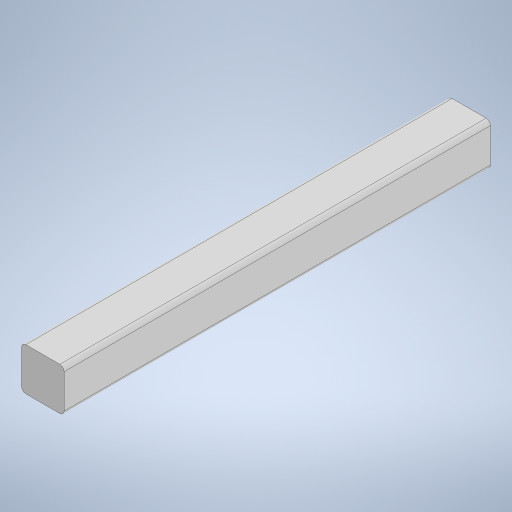
# Autodesk Inventor part: MagnetShaft
Saved by Autodesk Inventor 2024.4 (Build 284460000, 460)
## iProperties
Created: 2025-12-17
Part Number: MagnetShaft
Material: Generic
Document SubType Name: Modeling
Designer: jonas
Density: 1 g/cm^3
Appearance: Default
Author: jonas
Autodesk Inventor part; units mm, degrees
ref_plane "YZ Plane" through (0, 0, 0) normal (1, 0, 0) x (0, 1, 0)
ref_plane "XZ Plane" through (0, 0, 0) normal (0, 1, 0) x (-1, 0, 0)
ref_plane "XY Plane" through (0, 0, 0) normal (0, 0, 1) x (1, 0, 0)
sketch "Sketch1" plane through (0, 0, 0) normal (0, 1, 0) x (-1, 0, 0)
  line L0 (2, 0) -> (18, 0)
  line L1 (20, -2) -> (20, -18)
  line L2 (18, -20) -> (2, -20)
  line L3 (0, -18) -> (0, -2)
  arc A0 (20, -2) -> (18, 0) centre (18, -2) ccw
  arc A1 (2, 0) -> (0, -2) centre (2, -2) ccw
  arc A2 (0, -18) -> (2, -20) centre (2, -18) ccw
  arc A3 (18, -20) -> (20, -18) centre (18, -18) ccw
  point P0 (0, 0)
  point P1 (20, -20)
  point P2 (20, 0)
  point P3 (0, -20)
  dimension "d0" = 20
  dimension "d1" = 20
  dimension "d4" = 2
  constraints: 8 end point, 8 point on circle, 8 point on line, 8 tangent, 4 centre point, 3 equal radius, 2 parallel, 1 horizontal, 1 perpendicular
  measures "d0" distance of point (0, -20) point (0, 0)
  measures "d1" distance of point (0, 0) point (20, 0)
  measures "d4" radius of A0
extrude "Extrusion1" add sketch "Sketch1" along normal blind 200
body "Solid1"
